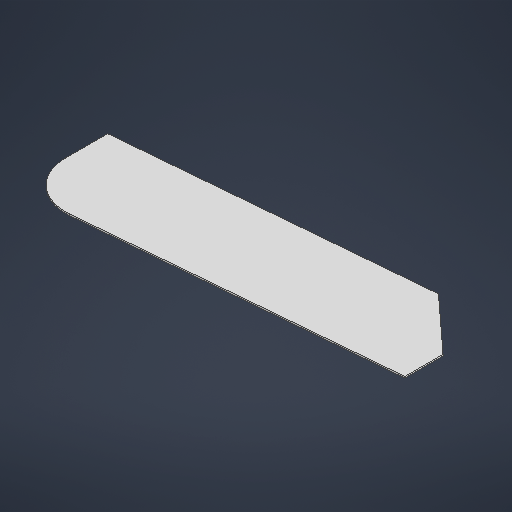
# Autodesk Inventor part: e
Saved by Autodesk Inventor 2027 (Build 310192000, 192)
## iProperties
Created: 2026-02-05
Part Number: e
Material: Generic
Document SubType Name: Modeling
Designer: Joefi
Density: 1 g/cm^3
Appearance: Default
Author: Joefi
Autodesk Inventor part; units mm, degrees
ref_plane "YZ Plane" through (0, 0, 0) normal (1, 0, 0) x (0, 1, 0)
ref_plane "XZ Plane" through (0, 0, 0) normal (0, 1, 0) x (-1, 0, 0)
ref_plane "XY Plane" through (0, 0, 0) normal (0, 0, 1) x (1, 0, 0)
sketch "Sketch1" plane through (0, 0, 0) normal (0, 1, 0) x (-1, 0, 0)
  line L0 (-0.7821, 21.3445) -> (84.5093, 28.8066)
  line L1 (84.5093, 28.8066) -> (84.5093, 40.7189)
  arc A0 (84.5093, 40.7189) -> (70.3763, 53.6694) centre (71.5093, 40.7189) ccw
  line L2 (70.3763, 53.6694) -> (-16.1101, 46.1028)
  line L3 (-16.1101, 46.1028) -> (-16.1101, 35.3901)
  line L4 (-16.1101, 35.3901) -> (-0.7821, 21.3445)
  line L5 (82.5093, 40.7189) -> (82.5093, 35.2209)
  arc A1 (77.9451, 30.2399) -> (82.5093, 35.2209) centre (77.5093, 35.2209) ccw
  line L6 (77.9451, 30.2399) -> (2.112, 23.6054)
  arc A2 (-1.7018, 24.8999) -> (2.112, 23.6054) centre (1.6762, 28.5863) ccw
  line L7 (-1.7018, 24.8999) -> (-12.4881, 34.7838)
  arc A3 (-14.1101, 38.4702) -> (-12.4881, 34.7838) centre (-9.1101, 38.4702) ccw
  line L8 (-14.1101, 38.4702) -> (-14.1101, 39.6885)
  arc A4 (-9.5459, 44.6695) -> (-14.1101, 39.6885) centre (-9.1101, 39.6885) ccw
  line L9 (-9.5459, 44.6695) -> (70.5506, 51.677)
  arc A5 (82.5093, 40.7189) -> (70.5506, 51.677) centre (71.5093, 40.7189) ccw
  line L10 (-15.9101, 45.9195) -> (70.3937, 53.4702)
  arc A6 (84.3093, 40.7189) -> (70.3937, 53.4702) centre (71.5093, 40.7189) ccw
  line L11 (84.3093, 40.7189) -> (84.3093, 28.9898)
  line L12 (84.3093, 28.9898) -> (-0.7118, 21.5514)
  line L13 (-0.7118, 21.5514) -> (-15.9101, 35.4781)
  line L14 (-15.9101, 35.4781) -> (-15.9101, 45.9195)
  point P0 (0, 0)
  dimension "d0" = 0.2
  constraints: 30 end point, 14 point on circle, 7 centre point, 5 other
  measures "d0" distance between parallel lines of L2 L10
extrude "Extrusion1" add sketch "Sketch1" along normal blind 0.4 contours L4 L3 L2 A0 L1 L0 | L5 A1 L6 A2 L7 A3 L8 A4 L9 A5 | L10 A6 L11 L12 L13 L14
body "Solid1"
